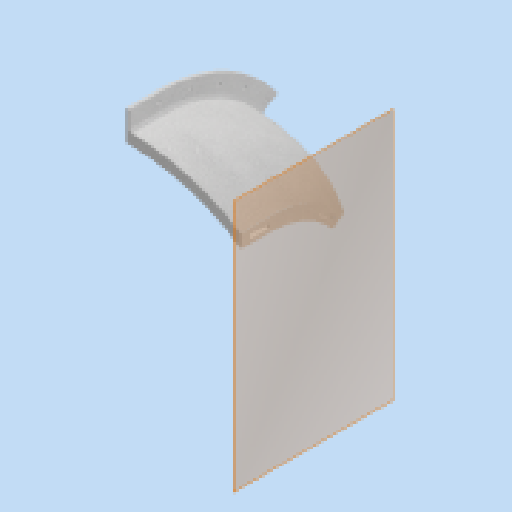
# Autodesk Inventor part: eggshellCorePrinted
Saved by Autodesk Inventor 2023 (Build 270158000, 158)
## iProperties
Created: 2026-03-19
Part Number: eggshellCorePrinted
Material: GFRC
Document SubType Name: Modeling
Designer: Nathann
Density: 1.7 g/cm^3
Appearance: Flat - Polished Gray
Mass: 25539 g
Surface Area: 11826.8 cm^2
Volume: 15023 cm^3
Author: Nathann
Autodesk Inventor part; units mm, degrees
ref_plane "XZ Plane" through (0, 0, 0) normal (0, 1, 0) x (-1, 0, 0)
ref_plane "XY Plane" through (0, 0, 0) normal (0, 0, 1) x (1, 0, 0)
sketch "Sketch1" plane through (0, 0, 0) normal (0, 0, 1) x (1, 0, 0)
  ellipse E0 centre (0, 0) end of major axis (0, 330) minor radius 450 (0, -330) -> (0, 330) ccw
  ellipse E1 centre (0, 0) end of major axis (420, 0) minor radius 300 (0, -300) -> (0, 300) ccw
  line L0 (0, 300) -> (0, 330)
  line L1 (0, -300) -> (0, -330)
  line L2 (420, 0) -> (450, 0)
  dimension "d0" = 420
  dimension "d1" = 450
  dimension "d2" = 300
  dimension "d3" = 330
  constraints: 6 end point, 2 coincident, 2 point on line, 1 horizontal, 10 other
extrude "Extrusion1" add sketch "Sketch1" along normal blind 80
sketch "Sketch2" plane through (0, 0, 80) normal (0, 0, 1) x (1, 0, 0)
  line L0 (0, 0) -> (451.5059, 0)
  ellipse E0 centre (0, 0) end of major axis (-450, 0) minor radius 330 (0, -330) -> (0, 330) ccw projected
  line L1 (0, 330) -> (0, 300) projected
  ellipse E1 centre (0, 0) end of major axis (-420, 0) minor radius 300 (0, -300) -> (0, 300) ccw projected
  line L2 (0, -300) -> (0, -330) projected
  point P0 (420, 0)
  point P1 (450, 0)
  constraints: 2 end point, 1 horizontal, 2 other
revolve "Revolution1" add sketch "Sketch2" angle 180 about axis through (0, 0, 80) along (1, 0, 0) contours E1 L1 E0 L0
sketch "Sketch3" plane through (0, 0, 0) normal (0, 0, -1) x (-1, 0, 0)
  ellipse E0 centre (0, 0) end of major axis (420, 0) minor radius 300 (0, 300) -> (0, -300) ccw projected
  line L0 (-410.6033, 63.104) -> (-375.8737, -133.8576)
  line L1 (-375.8737, -133.8576) -> (-428.5073, -143.1383)
  line L2 (-428.5073, -143.1383) -> (-456.291, 14.4309)
  line L3 (0, 300) -> (0, -300) projected
  ellipse E1 centre (0, 0) end of major axis (450, 0) minor radius 330 (0, 330) -> (0, -330) ccw projected
  line L4 (-456.291, 14.4309) -> (-439.6592, 70.3382)
  line L5 (-428.5073, -143.1383) -> (-336.4493, -219.1451)
  line L6 (-336.4493, -219.1451) -> (-375.8737, -133.8576)
  line L7 (-410.6033, 63.104) -> (-439.6592, 70.3382)
  line L8 (-393.2385, -35.3768) -> (260.9914, 90.2506)
  line L9 (260.9914, 90.2506) -> (260.9914, 44.7879)
  line L10 (260.9914, 44.7879) -> (0, 40.1342)
  dimension "d8" = 200
  dimension "d9" = 10
  dimension "d12" = 45.4627
  dimension "d13" = 160
  constraints: 20 end point, 2 perpendicular, 2 point on line, 1 midpoint, 1 vertical, 9 other
  measures "d8" distance of L0.start L0.end
  measures "d9" angle of L3 L0
  measures "d12" distance of L8.end L9.end
  measures "d13" distance of L1.end L2.end
extrude "Extrusion2" add sketch "Sketch3" against normal blind 160 contours L0 E0
ref_plane "Work Plane1" through (440.1475, 57.8945, 0) normal (-0.9848078, 0.1736482, 0) x (0, 0, 1)
sketch "Sketch5" plane through (440.1475, 57.8945, 0) normal (-0.9848078, 0.1736482, 0) x (0, 0, 1)
  line L0 (80, -458.4323) -> (80, -55.3041) projected
  circle A0 centre (80, -117.2866) radius 241.1725
  point P0 (0, -133.4458)
  constraints: 1 centre point, 1 point on line
extrude "Extrusion4" cut sketch "Sketch5" against normal blind 160
sketch "Sketch6" plane through (0, -330, 0) normal (-1, 0, 0) x (0, 0, 1)
  line L0 (0, 30) -> (0, 0) projected
  line L1 (0, 0) -> (80, 0) projected
  arc A0 (80, 0) -> (80, 660) centre (80, 330) ccw projected
  line L2 (0, 660) -> (80, 660) projected
  line L3 (0, 660) -> (0, 630) projected
  line L4 (0, 630) -> (80, 630) projected
  arc A1 (80, 30) -> (80, 630) centre (80, 330) ccw projected
  line L5 (0, 30) -> (80, 30) projected
  arc A2 (80, -50) -> (80, 710) centre (80, 330) ccw
  line L6 (80, -50) -> (-50, -50)
  line L7 (-50, -50) -> (-50, 80)
  line L8 (-50, 80) -> (80, 80)
  arc A3 (80, 80) -> (80, 580) centre (80, 330) ccw
  line L9 (80, 580) -> (-50, 580)
  line L10 (-50, 580) -> (-50, 710)
  line L11 (-50, 710) -> (80, 710)
  line L12 (0, 660) -> (0, 710)
  line L13 (0, 0) -> (0, -50)
  line L14 (80, 330) -> (410, 330)
  circle A4 centre (435, 330) radius 4.25
  circle A5 centre (426.0994, 408.9949) radius 4.25
  circle A6 centre (399.844, 484.0287) radius 4.25
  circle A7 centre (357.5502, 551.3389) radius 4.25
  circle A8 centre (301.3389, 607.5502) radius 4.25
  circle A9 centre (234.0288, 649.8439) radius 4.25
  circle A10 centre (158.995, 676.0994) radius 4.25
  circle A11 centre (80, 685) radius 4.25
  circle A12 centre (435, 330) radius 4.25
  circle A13 centre (426.0994, 251.0051) radius 4.25
  circle A14 centre (399.844, 175.9713) radius 4.25
  circle A15 centre (357.5502, 108.6611) radius 4.25
  circle A16 centre (301.3389, 52.4498) radius 4.25
  circle A17 centre (234.0288, 10.1561) radius 4.25
  circle A18 centre (158.995, -16.0994) radius 4.25
  circle A19 centre (80, -25) radius 4.25
  point P0 (0, 330)
  point P1 (460, 330)
  point P2 (80, -50)
  point P3 (460, 330)
  point P4 (439.25, 330)
  point P5 (430.75, 330)
  dimension "d19" = 50
  dimension "d22" = 8.5
  dimension "d25" = 90
  dimension "d27" = 25
  dimension "d28" = 0
  constraints: 18 centre point, 18 end point, 10 symmetric about line, 6 point on circle, 3 point on line, 1 perpendicular, 30 other
  measures "d19" distance between parallel lines of L1 L6
  measures "d22" diameter of A4
  measures "d27" distance of point (460, 330) A4.centre
  measures "d28" vertical distance of point (460, 330) A4.centre
extrude "Extrusion5" add sketch "Sketch6" against normal blind 10 contours L5 A1 L14 A0 L1 L0 | L1 A0 L2 L12 L11 A2 L6 L13 | A1 L4 L3 L2 A0 L14
ref_plane "Work Plane2" through (0, 0, 0) normal (0, 0, -1) x (-1, 0, 0)
mirror "Mirror1" about plane through (0, 0, 0) normal (0, 0, -1) of "Extrusion5", "Extrusion4", "Extrusion2", "Revolution1", "Extrusion1"
sketch "Sketch7" plane through (0, 0, 0) normal (0, 0, -1) x (-1, 0, 0)
  line L0 (-663.6694, -741.8919) -> (123.4449, -741.8919)
  line L1 (123.4449, -741.8919) -> (123.4449, 592.7802)
  line L2 (123.4449, 592.7802) -> (-663.6694, 592.7802)
  line L3 (-663.6694, 592.7802) -> (-663.6694, -741.8919)
  point P0 (0, 0)
  constraints: 8 end point, 2 parallel, 1 horizontal, 1 perpendicular
extrude "Extrusion6" cut sketch "Sketch7" against normal blind 1000
sketch "Sketch8" plane through (440.1475, 57.8945, 0) normal (0.9848078, -0.1736482, 0) x (0, 0, -1)
  line L0 (0, 6.7266) -> (80, 6.7266) projected
  line L1 (80, -205.7359) -> (0, -205.7359) projected
  circle A0 centre (80, -125.7359) radius 35
  line L2 (0, 6.7266) -> (0, -205.7359) projected
  circle A1 centre (80, -180.7359) radius 4.5
  circle A2 centre (118.8909, -164.6268) radius 4.5
  circle A3 centre (135, -125.7359) radius 4.5
  circle A4 centre (118.8909, -86.845) radius 4.5
  circle A5 centre (80, -70.7359) radius 4.5
  circle A6 centre (41.1091, -86.845) radius 4.5
  circle A7 centre (25, -125.7359) radius 4.5
  circle A8 centre (41.1091, -164.6268) radius 4.5
  point P0 (80.0002, -99.5046)
  dimension "d42" = 80
  dimension "d43" = 70
  dimension "d44" = 80
  dimension "d45" = 9
  dimension "d46" = 55
  dimension "d49" = 360
  constraints: 9 centre point, 1 vertical alignment, 17 other
  measures "d42" distance from line of L2 A0.centre
  measures "d43" diameter of A0
  measures "d44" distance from line of L1 A0.centre
  measures "d45" diameter of A1
  measures "d46" distance of A0.centre A1.centre
extrude "Extrusion7" cut sketch "Sketch8" against normal blind 50
ref_plane "Work Plane4" through (300, 0, 0) normal (1, 0, 0) x (0, 1, 0)
sketch "Sketch10" plane through (300, 0, 0) normal (1, 0, 0) x (0, 1, 0)
  line L0 (-646.9693, -896.2791) -> (523.3446, -896.2791)
  line L1 (523.3446, -896.2791) -> (523.3446, 327.6055)
  line L2 (523.3446, 327.6055) -> (-646.9693, 327.6055)
  line L3 (-646.9693, 327.6055) -> (-646.9693, -896.2791)
  point P0 (0, 0)
  constraints: 8 end point, 2 parallel, 1 horizontal, 1 perpendicular
extrude "Extrusion9" cut sketch "Sketch10" along normal through all
sketch "Sketch11" plane through (300, 0, 0) normal (1, 0, 0) x (0, 1, 0)
  line L0 (0, 0) -> (-527.7941, -914.1662)
  line L1 (0, 0) -> (515.8828, -893.5353)
  line L2 (515.8828, -893.5353) -> (-527.7941, -914.1662)
  line L3 (-641.389, 0) -> (573.3982, 0)
  line L4 (0, 0) -> (0, 166.7871)
  line L5 (515.8828, -893.5353) -> (515.8828, 0)
  line L6 (-527.7941, -914.1662) -> (-527.7941, 0)
  dimension "d59" = 60
  dimension "d60" = 60
  constraints: 14 end point, 3 point on line, 2 perpendicular, 1 horizontal, 1 vertical, 1 other
  measures "d59" angle of L0 L3
  measures "d60" angle of L3 L1
extrude "Extrusion10" cut sketch "Sketch11" against normal through all contours L1 L2 L0 | L0 L6 L3
sketch "Sketch12" plane through (300, 0, 0) normal (1, 0, 0) x (0, 0, -1)
  line L0 (25, 230.9675) -> (75, 230.9675)
  line L1 (75, 230.9675) -> (75, 220.9675)
  line L2 (75, 220.9675) -> (25, 220.9675)
  line L3 (25, 220.9675) -> (25, 230.9675)
  line L4 (0, 209.9563) -> (0, 245.9675) projected
  line L5 (0, 245.9675) -> (80, 245.9675) projected
  line L6 (241.1863, 153.2012) -> (202.884, 185.3406)
  line L7 (202.884, 185.3406) -> (209.3119, 193.001)
  line L8 (209.3119, 193.001) -> (247.6141, 160.8617)
  line L9 (247.6141, 160.8617) -> (241.1863, 153.2012)
  line L10 (238.1048, 188.422) -> (300.0063, 136.4806)
  point P0 (0, 0)
  dimension "d61" = 50
  dimension "d62" = 10
  dimension "d63" = 25
  dimension "d64" = 15
  dimension "d65" = 50
  dimension "d66" = 10
  dimension "d67" = 40
  dimension "d68" = 15
  dimension "d69" = 25
  constraints: 18 end point, 5 parallel, 2 perpendicular, 1 horizontal, 3 other
  measures "d61" distance of L1.end L2.end
  measures "d62" distance of L2.end L0.start
  measures "d63" distance between parallel lines of L4 L3
  measures "d64" distance between parallel lines of L5 L0
  measures "d65" distance of L7.end L8.end
  measures "d66" distance of L6.end L7.end
  measures "d67" angle of L5 L10
  measures "d68" distance between parallel lines of L10 L8
  measures "d69" distance from line of L9 L10.start
extrude "Extrusion11" cut sketch "Sketch12" against normal blind 15
fillet "Fillet1" radius 10 2 edges at (10, 295.2089, -227.3022) (10, 329.9185, -40)
fillet "Fillet2" radius 2 12 edges at (10, 338.6462, -252.3913) (10, 380, -40) (0, 380, -40) (0, 338.6462, -252.3913) (5, 380, 0) (12.8164, 332.7224, 0) (169.7256, 305.6278, 0) (10, 359.8396, 0) (162.7048, 276.5745, 0) (0, 340, 0) (0, 300, -40) (0, 269.2494, -212.3055)
sketch "Sketch13" plane through (300, 155.9876, -270.1785) normal (0, -0.8660254, -0.5) x (1, 0, 0)
  line L0 (-275, -72.3068) -> (-225, -72.3068)
  line L1 (-225, -72.3068) -> (-225, -62.3068)
  line L2 (-225, -62.3068) -> (-275, -62.3068)
  line L3 (-275, -62.3068) -> (-275, -72.3068)
  line L4 (-300, -133.1844) -> (-300, -56.6426) projected
  line L5 (-292, -137.3068) -> (-298, -137.3068)
  point P0 (-300, 311.9753)
  dimension "d74" = 50
  dimension "d75" = 10
  dimension "d76" = 25
  dimension "d77" = 65
  constraints: 10 end point, 2 horizontal, 2 parallel, 1 perpendicular, 2 other
  measures "d74" distance of L0.start L0.end
  measures "d75" distance of L0.end L1.end
  measures "d76" distance between parallel lines of L4 L3
  measures "d77" distance between parallel lines of L5 L0
extrude "Extrusion12" cut sketch "Sketch13" against normal blind 20
equation "\"d27\" = 0.5 * d19"
body "Solid1"
